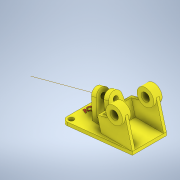
# Autodesk Inventor part: Reper_GoleaCristian
Saved by Autodesk Inventor 2021 (Build 250183000, 183)
## iProperties
Created: 2021-03-03
Part Number: Reper_GoleaCristian
Material: Steel, Carbon
Document SubType Name: Modeling
Designer: Crist
Density: 7.85 g/cm^3
Appearance: Canary
Mass: 882.333 g
Surface Area: 390.46 cm^2
Volume: 112.399 cm^3
Author: Crist
Autodesk Inventor part; units mm, degrees
ref_plane "YZ Plane" through (0, 0, 0) normal (1, 0, 0) x (0, 1, 0)
ref_plane "XZ Plane" through (0, 0, 0) normal (0, 1, 0) x (-1, 0, 0)
ref_plane "XY Plane" through (0, 0, 0) normal (0, 0, 1) x (1, 0, 0)
sketch "Sketch1" plane through (0, 0, 0) normal (0, 0, 1) x (1, 0, 0)
  line L0 (-29.4372, -7.8877) -> (176.6233, 47.3261) projected
  line L1 (101.2142, 39.5436) -> (109.9075, 41.8729)
  line L2 (109.9075, 41.8729) -> (118.9662, 8.0655)
  line L3 (118.9662, 8.0655) -> (132.4891, 11.689)
  line L4 (132.4891, 11.689) -> (123.4305, 45.4964)
  line L5 (123.4305, 45.4964) -> (132.1238, 47.8258)
  line L6 (132.1238, 47.8258) -> (144.9387, 0)
  line L7 (144.9387, 0) -> (111.8098, 0)
  line L8 (111.8098, 0) -> (101.2142, 39.5436)
  line L9 (-28.9877, 0) -> (173.9264, 0) projected
  point P0 (0, 0)
  dimension "d6" = 9
  dimension "d7" = 14
  dimension "d8" = 9
  dimension "d9" = 12
  dimension "d10" = 35
  dimension "d11" = 117
  constraints: 16 end point, 4 perpendicular, 2 point on line, 1 collinear, 1 horizontal, 1 parallel
  measures "d6" distance between parallel lines of L2 L8
  measures "d7" distance between parallel lines of L4 L2
  measures "d8" distance between parallel lines of L6 L4
  measures "d9" distance between parallel lines of L0 L5
  measures "d10" distance between parallel lines of L3 L1
  measures "d11" distance from line of point (0, 0) L2
extrude "Extrusion1" add sketch "Sketch1" along normal mid plane 50 contours L8 L1 L2 L0 | L0 L2 L3 L4 L6 L7 L8 | L4 L5 L6 L0
sketch "Sketch2" plane through (111.8098, 0, -25) normal (-0.9659258, -0.258819, 0) x (0, 0, 1)
  line L0 (25, 64.8401) -> (25, -46.4712) projected
  line L1 (13.2622, 31.4335) -> (1.57, -23.5744)
  line L2 (1.57, -23.5744) -> (48.43, -23.5744)
  line L3 (48.43, -23.5744) -> (36.7378, 31.4335)
  arc A0 (36.7378, 31.4335) -> (13.2622, 31.4335) centre (25, 28.9385) ccw
  line L4 (0, 40.9385) -> (50, 40.9385) projected
  line L5 (0, -8.5744) -> (50, -8.5744) projected
  dimension "d14" = 78
  dimension "d15" = 78
  dimension "d16" = 15
  constraints: 6 end point, 3 tangent, 2 point on circle, 1 centre point, 1 coincident, 1 horizontal
  measures "d14" angle of L2 L1
  measures "d15" angle of L3 L2
  measures "d16" distance between parallel lines of L5 L2
extrude "Extrusion2" cut sketch "Sketch2" against normal blind 50 keep common part
sketch "Sketch4" plane through (0, 0, 0) normal (0, 0, 1) x (1, 0, 0)
  line L0 (-28.9877, 0) -> (173.9264, 0) projected
  line L1 (-29.4372, -7.8877) -> (176.6233, 47.3261) projected
  line L2 (132.9832, 25.3) -> (156.1654, 31.5117)
  line L3 (156.1654, 31.5117) -> (153.5822, 41.1522)
  line L4 (153.5822, 41.1522) -> (182.56, 48.9168)
  line L5 (182.56, 48.9168) -> (195.6672, 0)
  line L6 (195.6672, 0) -> (139.7623, 0)
  line L7 (139.7623, 0) -> (132.9832, 25.3)
  line L8 (134.5839, 38.6446) -> (144.9387, 0) projected
  point P0 (0, 0)
  point P1 (195.6672, 0)
  dimension "d19" = 49
  dimension "d20" = 30
  dimension "d21" = 25.3
  dimension "d22" = 5
  constraints: 12 end point, 4 perpendicular, 2 collinear, 1 horizontal
  measures "d19" distance between parallel lines of L8 L5
  measures "d20" distance between parallel lines of L5 L3
  measures "d21" distance from line of L2.start L0
  measures "d22" distance between parallel lines of L8 L7
extrude "Extrusion3" add sketch "Sketch4" along normal mid plane 61 contours L7 L2 L8 L0 | L8 L2 L3 L1 L4 L5 L6 L0
sketch "Sketch5" plane through (153.5822, 41.1522, 30.5) normal (-0.258819, 0.9659258, 0) x (0.9659258, 0.258819, 0)
  line L0 (-19, 56) -> (35, 56)
  line L1 (35, 56) -> (35, 5)
  line L2 (35, 5) -> (-19, 5)
  line L3 (-19, 5) -> (-19, 56)
  line L4 (30, 61) -> (30, 0) projected
  line L5 (-24, 0) -> (-24, 16.1105) projected
  line L6 (30, 0) -> (0, 0) projected
  line L7 (0, 61) -> (30, 61) projected
  point P0 (-159, 30.5)
  dimension "d25" = 5
  dimension "d26" = 5
  dimension "d27" = 5
  dimension "d28" = 5
  constraints: 8 end point, 2 parallel, 1 horizontal, 1 perpendicular
  measures "d25" distance between parallel lines of L1 L4
  measures "d26" distance between parallel lines of L5 L3
  measures "d27" distance between parallel lines of L6 L2
  measures "d28" distance between parallel lines of L7 L0
extrude "Extrusion4" cut sketch "Sketch5" against normal through all
sketch "Sketch6" plane through (0, 0, 0) normal (0, 0, 1) x (1, 0, 0)
  line L0 (153.5822, 41.1522) -> (182.56, 48.9168) projected
  circle A0 centre (168.0711, 45.0345) radius 15
  line L1 (182.56, 48.9168) -> (195.6672, 0) projected
  point P0 (0, 0)
  constraints: 1 centre point, 1 midpoint, 1 tangent
extrude "Extrusion5" add sketch "Sketch6" along normal mid plane 71
sketch "Sketch7" plane through (0, 0, 0) normal (0, 0, 1) x (1, 0, 0)
  circle A0 centre (168.0711, 45.0345) radius 19.5
  circle A1 centre (168.0711, 45.0345) radius 15 projected
  point P0 (0, 0)
  dimension "d36" = 39
  constraints: 1 centre point, 1 concentric
  measures "d36" diameter of A0
extrude "Extrusion6" cut sketch "Sketch7" against normal mid plane 41 contours A0 | A1
sketch "Sketch8" plane through (0, 0, 0) normal (0, 1, 0) x (-1, 0, 0)
  line L0 (-82.6672, -35) -> (-82.6672, 35)
  line L1 (-91.6172, 42.9434) -> (-195.6672, 30.5)
  line L2 (-195.6672, 30.5) -> (-195.6672, -30.5)
  line L3 (-195.6672, -30.5) -> (-91.6172, -42.9434)
  arc A0 (-91.6172, -42.9434) -> (-82.6672, -35) centre (-90.6672, -35) ccw
  arc A1 (-82.6672, 35) -> (-91.6172, 42.9434) centre (-90.6672, 35) ccw
  line L4 (39.1334, 0) -> (-234.8006, 0) projected
  point P0 (0, 0)
  dimension "d39" = 8
  dimension "d40" = 113
  dimension "d41" = 70
  dimension "d42" = 35
  constraints: 8 end point, 4 point on circle, 4 tangent, 2 centre point, 1 coincident, 1 equal radius, 1 parallel, 1 vertical
  measures "d39" radius of A0
  measures "d40" distance between parallel lines of L2 L0
  measures "d41" distance of A0.centre A1.centre
  measures "d42" distance from line of A1.centre L4
extrude "Extrusion7" add sketch "Sketch8" against normal blind 6
sketch "Sketch12" plane through (168.0711, 45.0345, 35.5) normal (0, 0, 1) x (1, 0, 0)
  circle A0 centre (0, 0) radius 15 projected
  point P0 (-168.0711, -45.0345)
  constraints: 1 coincident
hole "Hole4" at (168.0711, 45.0345, 35.5) direction (0, 0, -1) diameter 15 end through all
sketch "Sketch13" plane through (104.32, 27.9525, 0) normal (-0.9659258, -0.258819, 0) x (0, 0, 1)
  arc A0 (11.7378, 2.4949) -> (-11.7378, 2.4949) centre (0, 0) ccw projected
  constraints: 1 coincident
hole "Hole5" at (104.32, 27.9525, 0) direction (0.9659258, 0.258819, 0) diameter 9 end through all
sketch "Sketch14" plane through (0, 0, 0) normal (0, 1, 0) x (1, 0, 0)
  arc A0 (91.6172, 42.9434) -> (82.6672, 35) centre (90.6672, 35) ccw projected
  point P0 (0, 0)
  constraints: 1 coincident
hole "Hole6" at (90.6672, 0, -35) direction (0, -1, 0) diameter 9 end through all
sketch "Sketch15" plane through (0, 0, 0) normal (0, 1, 0) x (1, 0, 0)
  arc A0 (82.6672, -35) -> (91.6172, -42.9434) centre (90.6672, -35) ccw projected
  point P0 (0, 0)
  constraints: 1 coincident
hole "Hole7" at (90.6672, 0, 35) direction (0, -1, 0) diameter 9 end through all
sketch "Sketch16" plane through (0, 0, 0) normal (0, 1, 0) x (1, 0, 0)
  line L0 (97.6672, 14.5) -> (97.6672, -14.5) construction
  line L1 (97.6672, -14.5) -> (86.6672, -14.5) construction
  line L2 (86.6672, -14.5) -> (86.6672, 14.5) construction
  line L3 (86.6672, 14.5) -> (97.6672, 14.5) construction
  line L4 (82.6672, 35) -> (82.6672, -35) projected
  spline S0 degree 2 poles (86.9646, 8.5697) (86.9646, 10.5875) (88.9095, 12.7593) (90.7896, 12.7593) knots 0 0 0 1 2 2 2
  line L5 (90.7896, 12.7593) -> (97.1753, 12.7593)
  line L6 (97.1753, 12.7593) -> (97.1753, 10.2472)
  line L7 (97.1753, 10.2472) -> (90.9354, 10.2472)
  spline S1 degree 2 poles (90.9354, 10.2472) (89.8901, 10.2472) (88.869, 9.4611) (88.869, 8.5697) knots 0 0 0 1 2 2 2
  spline S2 degree 2 poles (88.869, 8.5697) (88.869, 7.7026) (89.8495, 6.8922) (90.9354, 6.8922) knots 0 0 0 1 2 2 2
  line L8 (90.9354, 6.8922) -> (97.1753, 6.8922)
  line L9 (97.1753, 6.8922) -> (97.1753, 4.3801)
  line L10 (97.1753, 4.3801) -> (90.7977, 4.3801)
  spline S3 degree 2 poles (90.7977, 4.3801) (88.95, 4.3801) (86.9646, 6.4951) (86.9646, 8.5697) knots 0 0 0 1 2 2 2
  spline S4 degree 2 poles (86.9808, -1.8598) (86.9808, 0.393) (89.7037, 3.0348) (92.1672, 3.0348) knots 0 0 0 1 2 2 2
  spline S5 degree 2 poles (92.1672, 3.0348) (94.5416, 3.0348) (97.3698, 0.3849) (97.3698, -1.8679) knots 0 0 0 1 2 2 2
  spline S6 degree 2 poles (97.3698, -1.8679) (97.3698, -2.4595) (97.232, -3.4157) (97.1186, -3.8533) knots 0 0 0 1 2 2 2
  spline S7 degree 2 poles (97.1186, -3.8533) (97.0132, -4.1937) (96.6648, -4.9959) (96.5351, -5.2472) knots 0 0 0 1 2 2 2
  line L11 (96.5351, -5.2472) -> (94.1526, -5.2472)
  line L12 (94.1526, -5.2472) -> (94.1526, -4.9959)
  spline S8 degree 2 poles (94.1526, -4.9959) (94.3147, -4.8096) (94.7685, -4.2585) (94.9792, -3.91) knots 0 0 0 1 2 2 2
  spline S9 degree 2 poles (94.9792, -3.91) (95.198, -3.5616) (95.4978, -2.7269) (95.4978, -2.265) knots 0 0 0 1 2 2 2
  spline S10 degree 2 poles (95.4978, -2.265) (95.4978, -1.722) (95.1575, -0.8225) (94.728, -0.4092) knots 0 0 0 1 2 2 2
  spline S11 degree 2 poles (94.728, -0.4092) (94.3471, -0.0365) (93.0424, 0.4417) (92.1591, 0.4417) knots 0 0 0 1 2 2 2
  spline S12 degree 2 poles (92.1591, 0.4417) (91.2272, 0.4417) (89.9549, -0.0527) (89.5659, -0.4579) knots 0 0 0 1 2 2 2
  spline S13 degree 2 poles (89.5659, -0.4579) (89.185, -0.8468) (88.8528, -1.8031) (88.8528, -2.2812) knots 0 0 0 1 2 2 2
  spline S14 degree 2 poles (88.8528, -2.2812) (88.8528, -2.7755) (89.185, -3.675) (89.3876, -3.983) knots 0 0 0 1 2 2 2
  spline S15 degree 2 poles (89.3876, -3.983) (89.5902, -4.3233) (90.0197, -4.8339) (90.1899, -5.0203) knots 0 0 0 1 2 2 2
  line L13 (90.1899, -5.0203) -> (90.1899, -5.2472)
  line L14 (90.1899, -5.2472) -> (87.8398, -5.2472)
  spline S16 degree 2 poles (87.8398, -5.2472) (87.7101, -4.9716) (87.386, -4.2504) (87.2725, -3.8614) knots 0 0 0 1 2 2 2
  spline S17 degree 2 poles (87.2725, -3.8614) (87.1267, -3.3914) (86.9808, -2.5729) (86.9808, -1.8598) knots 0 0 0 1 2 2 2
  line L15 (94.7199, -13.6507) -> (87.1753, -10.9441)
  line L16 (87.1753, -10.9441) -> (87.1753, -8.3752)
  line L17 (87.1753, -8.3752) -> (94.7199, -5.6929)
  line L18 (94.7199, -5.6929) -> (94.7199, -8.1645)
  line L19 (94.7199, -8.1645) -> (89.7361, -9.7042)
  line L20 (89.7361, -9.7042) -> (94.7199, -11.2277)
  line L21 (94.7199, -11.2277) -> (94.7199, -13.6507)
  point P0 (0, 0)
  point P1 (86.6672, 0)
  point P2 (82.6672, 0)
  dimension "d94" = 15
  dimension "d95" = 29
  dimension "d96" = 11
  constraints: 2 midpoint, 1 horizontal alignment, 1 parallel, 2 other
  measures "d94" distance between parallel lines of L4 L0
  measures "d95" distance between parallel lines of L1 L3
  measures "d96" distance between parallel lines of L0 L2
emboss "Emboss1" sketch "Sketch16" operation add depth 1 direction (0, -1, 0)
equation "\"d15\" = d14"
equation "\"d36\" = 1.3 * d20"
equation "\"d42\" = 0.5 * d41"
body "Solid1"
